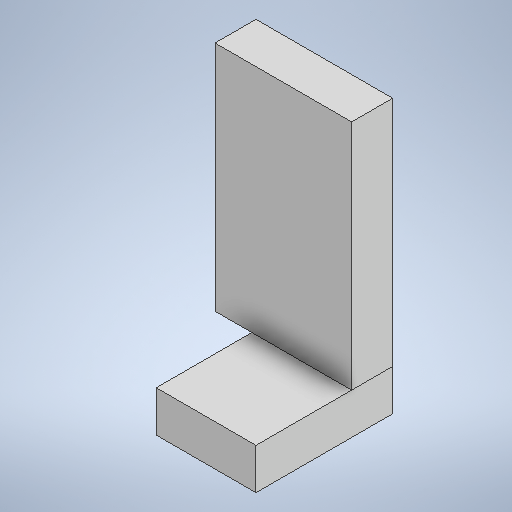
# Autodesk Inventor part: Eckverbinder_20x20
Saved by Autodesk Inventor 2025 (Build 290162000, 162)
## iProperties
Created: 2026-06-23
Part Number: Eckverbinder_20x20
Material: Generisch
Document SubType Name: Modeling
Designer: GemmiDad-GBSE
Density: 1 g/cm^3
Appearance: Vorgabe
Author: GemmiDad-GBSE
Autodesk Inventor part; units mm, degrees
ref_plane "YZ Plane" through (0, 0, 0) normal (1, 0, 0) x (0, 1, 0)
ref_plane "XZ Plane" through (0, 0, 0) normal (0, 1, 0) x (-1, 0, 0)
sketch "Skizze1" plane through (0, 0, 0) normal (0, 0, 1) x (1, 0, 0)
  line L0 (0, 0) -> (10, 0)
  line L1 (10, 0) -> (10, 10)
  line L2 (10, 10) -> (0, 10)
  line L3 (0, 10) -> (0, 0)
  constraints: 8 end point, 2 parallel, 1 horizontal, 1 perpendicular
extrude "Extrusion1" add sketch "Skizze1" along normal blind 3
ref_plane "Arbeitsebene1" through (0, 0, 3) normal (0, 0, 1) x (1, 0, 0)
sketch "Skizze2" plane through (0, 0, 3) normal (0, 0, 1) x (1, 0, 0)
  line L0 (0, 7) -> (10, 7)
  line L1 (10, 7) -> (10, 10)
  line L2 (10, 10) -> (0, 10)
  line L3 (0, 10) -> (0, 7)
  constraints: 8 end point, 2 parallel, 1 horizontal, 1 perpendicular
extrude "Extrusion2" add sketch "Skizze2" along normal blind 17 separate body
sketch "Skizze3" plane through (0, 0, 0) normal (0, 0, 1) x (1, 0, 0)
  circle A0 centre (0, 0) radius 2.7
  circle A1 centre (0, 5) radius 2.7
  constraints: 2 centre point
extrude "Extrusion3" cut sketch "Skizze3" along normal blind 3 bodies 1
sketch "Skizze4" plane through (0, 0, 0) normal (0, 1, 0) x (-1, 0, 0)
  circle A0 centre (0, 3) radius 2.7
  constraints: 1 centre point
extrude "Extrusion4" cut sketch "Skizze4" along normal mid plane 20 bodies 1
